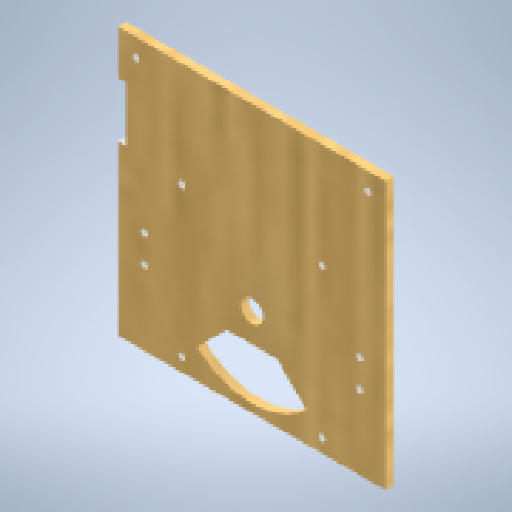
# Autodesk Inventor part: Madera intermedia
Saved by Autodesk Inventor 2023 (Build 270158000, 158)
## iProperties
Created: 2022-12-03
Part Number: Madera intermedia
Material: Genérico
Document SubType Name: Modeling
Designer: sergi
Density: 1 g/cm^3
Appearance: Valor por defecto
Author: sergi
Autodesk Inventor part; units mm, degrees
ref_plane "YZ Plane" through (0, 0, 0) normal (1, 0, 0) x (0, 1, 0)
ref_plane "XZ Plane" through (0, 0, 0) normal (0, 1, 0) x (-1, 0, 0)
ref_plane "XY Plane" through (0, 0, 0) normal (0, 0, 1) x (1, 0, 0)
sketch "Boceto1" plane through (0, 0, 0) normal (0, 0, 1) x (1, 0, 0)
  line L0 (48.5, -35) -> (48.5, 68) projected
  line L1 (48.5, 65) -> (35.5, 65) projected
  line L2 (-48.5, 68) -> (-48.5, -35) projected
  line L3 (-48.5, -32) -> (48.5, -32) projected
  line L4 (-48.5, -32) -> (48.5, -32)
  line L5 (48.5, -32) -> (48.5, 65)
  line L6 (48.5, 65) -> (-48.5, 65)
  line L7 (-48.5, 65) -> (-48.5, -32)
  point P0 (0, 0)
  point P1 (-48.5, 65)
  constraints: 8 end point, 2 parallel, 1 horizontal, 1 perpendicular, 1 other
extrude "Extrusión1" add sketch "Boceto1" along normal blind 3
sketch "Boceto5" plane through (0, 0, 0) normal (0, 0, -1) x (-1, 0, 0)
  line L0 (11.3801, -12.7901) -> (-11.3717, -12.7901)
  line L1 (19.791, -21.201) -> (5.6217, -7.0317) projected
  line L2 (-5.6132, -7.0317) -> (-19.7826, -21.201) projected
  line L3 (9.0613, -10.4713) -> (-9.0529, -10.4713)
  arc A0 (-19.7826, -21.201) -> (19.791, -21.201) centre (0.0042, 0) ccw projected
  point P0 (0, 0)
  constraints: 4 end point, 4 point on line
extrude "Extrusión5" cut sketch "Boceto5" against normal through all
sketch "Boceto6" plane through (0, 0, 0) normal (0, 0, -1) x (-1, 0, 0)
  arc A0 (-19.7826, -21.201) -> (19.791, -21.201) centre (0.0042, 0) ccw projected
  circle A1 centre (-38.9983, 5) radius 1.25 projected
  circle A2 centre (-38.9983, 5) radius 1.25 projected
  circle A3 centre (-38.9983, -5) radius 1.25 projected
  circle A4 centre (39.0017, 5) radius 1.25 projected
  circle A5 centre (39.0017, 5) radius 1.25 projected
  circle A6 centre (39.0017, -5) radius 1.25 projected
  point P0 (0, 0)
  constraints: 1 coincident
hole "Agujero1" at (-0.0042, 0, 0) direction (0, 0, 1) diameter 8.1 end through all
sketch "Boceto7" plane through (0, 0, 0) normal (0, 0, -1) x (-1, 0, 0)
  circle A0 centre (25.3722, 27.0019) radius 1.5 projected
  circle A1 centre (0.0042, 0) radius 4.05 projected
  arc A2 (-19.7826, -21.201) -> (19.791, -21.201) centre (0.0042, 0) ccw projected
  line L0 (-19.7826, -21.201) -> (-9.0529, -10.4713) projected
  line L1 (-9.0529, -10.4713) -> (9.0613, -10.4713) projected
  line L2 (9.0613, -10.4713) -> (19.791, -21.201) projected
  line L3 (48.5, 65) -> (48.5, -32) projected
  line L4 (-48.5, 65) -> (48.5, 65) projected
  line L5 (-48.5, -32) -> (-48.5, 65) projected
  line L6 (48.5, -32) -> (-48.5, -32) projected
  circle A3 centre (-25.3678, 26.9981) radius 1.5 projected
  circle A4 centre (-25.3638, -27.0019) radius 1.25 projected
  circle A5 centre (25.3762, -26.9981) radius 1.25 projected
  circle A6 centre (-42, 58.5) radius 1.25 projected
  circle A7 centre (42, 58.5) radius 1.25 projected
  circle A8 centre (-38.9983, 5) radius 1.25 projected
  circle A9 centre (-38.9983, 5) radius 1.25 projected
  circle A10 centre (-38.9983, -5) radius 1.25 projected
  circle A11 centre (39.0017, -5) radius 1.25 projected
  circle A12 centre (39.0017, 5) radius 1.25 projected
  point P0 (0, 0)
hole "Agujero2" at (-25.3762, -26.9981, 0) at (25.3638, -27.0019, 0) at (25.3678, 26.9981, 0) at (-25.3722, 27.0019, 0) at (42, 58.5, 0) at (-42, 58.5, 0) at (38.9983, -5, 0) at (38.9983, 5, 0) at (-39.0017, -5, 0) at (-39.0017, 5, 0) direction (0, 0, 1) diameter 2.5 end through all
sketch "Boceto9" plane through (0, 0, 0) normal (0, 0, -1) x (-1, 0, 0)
  line L0 (48.5, 65) -> (48.5, 49)
  line L1 (48.5, 65) -> (48.5, -32) projected
  line L2 (48.5, 49) -> (45.5, 49)
  line L3 (45.5, 49) -> (45.5, 29)
  line L4 (45.5, 29) -> (48.5, 29)
  point P0 (0, 0)
  dimension "d32" = 16
  dimension "d33" = 3
  dimension "d34" = 20
  constraints: 8 end point, 2 perpendicular, 2 point on line, 1 horizontal
  measures "d32" distance of L0.start L0.end
  measures "d33" distance of L0.end L2.end
  measures "d34" distance of L2.end L3.end
extrude "Extrusión7" cut sketch "Boceto9" against normal blind 10
